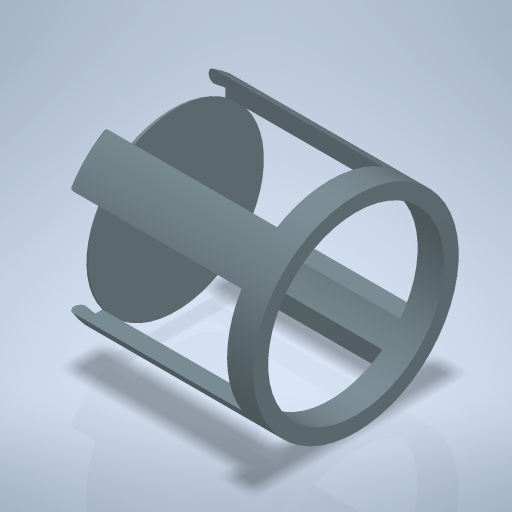
# Autodesk Inventor part: frame
Saved by Autodesk Inventor 2024 (Build 280153000, 153)
## iProperties
Created: 2024-04-24
Part Number: frame
Material: Blei
Document SubType Name: Modeling
Designer: ffogue
Density: 11.34 g/cm^3
Appearance: Blei
Author: ffogue
Autodesk Inventor part; units mm, degrees
ref_plane "YZ Plane" through (0, 0, 0) normal (1, 0, 0) x (0, 1, 0)
sketch "Skizze1" plane through (0, 0, 0) normal (0, 1, 0) x (1, 0, 0)
  line L0 (0, 19.5) -> (35, 19.5)
  line L1 (35, 19.5) -> (35, 0)
  line L2 (0, 0) -> (35, 0)
  line L3 (0.2, 0) -> (0.2, 18)
  line L4 (0.2, 18) -> (-1.7741, 17.5275)
  arc A0 (-2.0069, 19.5) -> (-1.7741, 17.5275) centre (-2.0069, 18.5) ccw
  line L5 (-2.0069, 19.5) -> (0, 19.5)
  point P0 (-3, 18.3828)
  dimension "d0" = 35
  dimension "d3" = 39
  dimension "d31" = 36
  dimension "d32" = 0.2
  dimension "d33" = 38
  dimension "d35" = 1
  dimension "d54" = 34.8
  constraints: 12 end point, 3 point on circle, 3 tangent, 2 perpendicular, 1 centre point, 1 coincident, 1 horizontal, 1 point on line, 1 vertical
  measures "d0" distance of L2.start L1.end
  measures "d3" diameter of L0.end L2
  measures "d31" diameter of L3.end L2
  measures "d32" distance from line of point (0, 0) L3
  measures "d33" horizontal distance of point (-3, 18.383) L0.end
  measures "d35" radius of A0
  measures "d54" distance between parallel lines of L1 L3
revolve "Umdrehung1" add sketch "Skizze1" angle 360 about axis through (0, 0, 0) along (1, 0, 0)
sketch "Skizze4" plane through (35, 0, 0) normal (1, 0, 0) x (0, 0, -1)
  circle A0 centre (0, 0) radius 16.7
  dimension "d18" = 33.4
  constraints: 1 centre point, 1 coincident
  measures "d18" diameter of A0
extrude "Extrusion2" cut sketch "Skizze4" against normal blind 34.2
ref_plane "Arbeitsebene2" through (0, 0, 19.5) normal (0, 0, 1) x (1, 0, 0)
sketch "Skizze5" plane through (0, 0, 19.5) normal (0, 0, 1) x (1, 0, 0)
  line L0 (0, 0) -> (42.5871, 0) construction
  line L1 (-0.5069, 10) -> (30, 10)
  line L2 (30, 10) -> (30, -10)
  line L3 (30, -10) -> (-0.5069, -10)
  line L4 (-0.5069, -10) -> (-0.5069, 10)
  line L5 (35, -19.5) -> (35, 19.5) projected
  line L6 (-2.0069, -19.5) -> (-2.0069, 19.5) projected
  dimension "d22" = 5
  dimension "d23" = 20
  dimension "d38" = 1.5
  constraints: 10 end point, 2 horizontal, 2 parallel, 1 perpendicular, 1 other
  measures "d22" distance between parallel lines of L2 L5
  measures "d23" distance between parallel lines of L3 L1
  measures "d38" distance between parallel lines of L6 L4
extrude "Extrusion5" cut sketch "Skizze5" against normal up to surface round surface about axis through (35, 0, 0) along (-1, 0, 0) radius 16.7 far side no
pattern_circular "Runde Anordnung3" count 4 over 360 about axis through (16.4966, 0, 0) along (1, 0, 0) of "Extrusion5"
ref_plane "Arbeitsebene5" through (0, 19.5, 0) normal (0, 1, 0) x (-1, 0, 0)
sketch "Skizze8" plane through (0, 19.5, 0) normal (0, 1, 0) x (-1, 0, 0)
  line L0 (-0.2, -10) -> (-0.8, -10) projected
  line L1 (-0.8, 10) -> (-0.2, 10) projected
  line L2 (3.0069, 18.5) -> (3.0069, -18.5) projected
  line L3 (3.0069, -10) -> (3.0069, 10)
  line L4 (3.0069, -10) -> (-0.8, -10)
  line L5 (-0.8, -10) -> (-0.8, 10) projected
  line L6 (0.5069, -10) -> (0.5069, 10) projected
  line L7 (-0.2, 10) -> (3.0069, 10)
  line L8 (-0.8, -10) -> (-0.2, 10)
  point P0 (0, 0)
  point P1 (0.5192, 10)
  constraints: 8 end point, 2 horizontal, 2 point on line
extrude "Extrusion8" cut sketch "Skizze8" against normal blind 10 contours L0 L8 L7 L6 L4 | L6 L7 L2 L4
pattern_circular "Runde Anordnung4" count 4 over 360 about axis through (-0.7871, 0, 0) along (1, 0, 0) of "Extrusion8"
